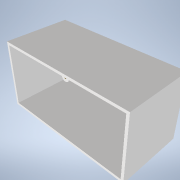
# Autodesk Inventor part: bottom
Saved by Autodesk Inventor 2021 (Build 250183000, 183)
## iProperties
Created: 2021-03-15
Part Number: bottom
Material: Všeobecné
Document SubType Name: Modeling
Designer: kanyk
Density: 1 g/cm^3
Appearance: Výchozí
Author: kanyk
Autodesk Inventor part; units mm, degrees
ref_plane "YZ Plane" through (0, 0, 0) normal (1, 0, 0) x (0, 1, 0)
ref_plane "XZ Plane" through (0, 0, 0) normal (0, 1, 0) x (-1, 0, 0)
ref_plane "XY Plane" through (0, 0, 0) normal (0, 0, 1) x (1, 0, 0)
sketch "Náčrt1" plane through (0, 0, 0) normal (0, 0, 1) x (1, 0, 0)
  line L0 (0, 0) -> (100, 0)
  line L1 (100, 0) -> (100, 50)
  line L2 (100, 50) -> (0, 50)
  line L3 (0, 50) -> (0, 0)
  dimension "d0" = 100
  dimension "d1" = 50
  constraints: 8 end point, 2 parallel, 1 horizontal, 1 perpendicular
  measures "d0" distance of L2.end L1.end
  measures "d1" distance of L1.end L0.end
extrude "Vysunutí1" add sketch "Náčrt1" along normal blind 49
sketch "Náčrt2" plane through (0, 0, 49) normal (0, 0, 1) x (1, 0, 0)
  line L0 (2, 2) -> (98, 2)
  line L1 (98, 2) -> (98, 48)
  line L2 (98, 48) -> (2, 48)
  line L3 (2, 48) -> (2, 2)
  point P0 (0, 0)
  dimension "d4" = 96
  dimension "d5" = 46
  constraints: 8 end point, 2 parallel, 1 horizontal, 1 perpendicular
  measures "d4" distance of L2.end L1.end
  measures "d5" distance of L1.end L0.end
extrude "Vysunutí2" cut sketch "Náčrt2" against normal blind 48
sketch "Náčrt3" plane through (0, 0, 1) normal (0, 0, 1) x (1, 0, 0)
  circle A0 centre (10, 10) radius 4
  line L0 (98, 48) -> (98, 2) projected
  line L1 (2, 48) -> (98, 48) projected
  line L2 (2, 2) -> (2, 48) projected
  line L3 (98, 2) -> (2, 2) projected
  circle A1 centre (10, 40) radius 4
  circle A2 centre (90, 10) radius 4
  circle A3 centre (90, 40) radius 4
  line L4 (98, 2) -> (2, 2) projected
  line L5 (50, 25) -> (2, 2)
  point P0 (0, 0)
  point P1 (10.387, 6.0188)
  point P2 (12.8605, 7.204)
  dimension "d8" = 8
  dimension "d11" = 30
  dimension "d14" = 80
  dimension "d19" = 25.602
  dimension "d20" = 40
  dimension "d22" = 15
  dimension "d23" = 48
  constraints: 4 centre point, 2 end point, 1 horizontal, 1 vertical, 6 other
  measures "d8" diameter of A0
  measures "d11" distance of A0.centre A1.centre
  measures "d14" distance of A0.centre A2.centre
  measures "d19" angle of L3 L5
  measures "d20" horizontal distance of L5.start A0.centre
  measures "d22" vertical distance of L5.start A0.centre
  measures "d23" horizontal distance of L2.start L5.start
extrude "Vysunutí3" add sketch "Náčrt3" along normal blind 10 contours A0 L5 | A1 | A2 | A3 picked at (11.6868, 9.0428)
hole "Díra1" at (10.0461, 9.9039, 11) direction (0, 0, -1) diameter 2.459 end through all thread size "M3x0.5" class "6H" standard "ISO Metric profile"
sketch "Náčrt4" plane through (0, 0, 0) normal (0, 0, -1) x (-1, 0, 0)
  point P0 (0, 0)
hole "Díra2" at (90, 40, 11) direction (0, 0, -1) diameter 2.459 end through all thread size "M3x0.5" class "6H" standard "ISO Metric profile"
hole "Díra3" at (90, 10, 11) direction (0, 0, -1) diameter 2.459 end through all thread size "M3x0.5" class "6H" standard "ISO Metric profile"
hole "Díra4" at (10, 40, 11) direction (0, 0, -1) diameter 2.459 end through all thread size "M3x0.5" class "6H" standard "ISO Metric profile"
equation "\"d22\" = 0.5 * d11"
